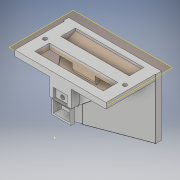
# Autodesk Inventor part: ventilador controladora
Saved by Autodesk Inventor 2019 (Build 230136000, 136)
## iProperties
Created: 2018-08-15
Part Number: ventilador controladora
Material: Genérico
Document SubType Name: Modeling
Designer: Albert Garangou Culebras
Density: 1 g/cm^3
Appearance: Valor por defecto
Author: Albert Garangou Culebras
Autodesk Inventor part; units mm, degrees
sketch "Boceto1" plane through (0, 0, 0) normal (0, 0, 1) x (1, 0, 0)
  line L0 (0, 0) -> (16, 0)
  line L1 (16, 0) -> (16, -12)
  line L2 (16, -12) -> (0, -12)
  line L3 (0, -12) -> (0, 0)
  line L4 (1, -1) -> (15, -1)
  line L5 (15, -1) -> (15, -11)
  line L6 (15, -11) -> (1, -11)
  line L7 (1, -11) -> (1, -1)
  dimension "d0" = 16
  dimension "d1" = 12
  constraints: 16 end point, 4 parallel, 2 horizontal, 2 perpendicular
  measures "d0" distance of L1.end L2.end
  measures "d1" distance of L0.end L1.end
ref_plane "Plano de trabajo3" through (0, 0, -40) normal (0, 0, -1) x (-1, 0, 0)
sketch "Boceto4" plane through (0, 0, -40) normal (0, 0, -1) x (-1, 0, 0)
  line L0 (0, -12) -> (0, 0) projected
  line L1 (0, -6) -> (-16, -6)
  line L2 (-8, -31) -> (-48, -31)
  line L3 (-8, -31) -> (32, -31)
  line L4 (32, -31) -> (32, 19)
  line L5 (32, 19) -> (-48, 19)
  line L6 (-48, 19) -> (-48, -31)
  dimension "d8" = 40
  dimension "d9" = 40
  dimension "d10" = 80
  constraints: 12 end point, 2 horizontal, 1 midpoint, 1 perpendicular, 1 vertical
  measures "d8" distance of L2.start L2.end
  measures "d9" distance of L2.start L3.end
  measures "d10" distance of L4.end L5.end
extrude "Extrusión2" add sketch "Boceto1" against normal blind 40
loft "Solevación1" add profiles "Boceto4" section 1 edges at (1, -6, 0) (8, -1, 0) (15, -6, 0) (8, -11, 0)
sketch "Boceto5" plane through (0, 0, -40) normal (0, 0, -1) x (-1, 0, 0)
  line L0 (30, -29) -> (-46, -29)
  line L1 (-46, -29) -> (-46, 17)
  line L2 (-46, 17) -> (30, 17)
  line L3 (30, 17) -> (30, -29)
  point P0 (0, 0)
  constraints: 8 end point, 2 parallel, 1 horizontal, 1 perpendicular
sketch "Boceto6" plane through (0, 0, 0) normal (0, 0, 1) x (1, 0, 0)
  line L0 (1, -11) -> (15, -11)
  line L1 (15, -11) -> (15, -1)
  line L2 (15, -1) -> (1, -1)
  line L3 (1, -1) -> (1, -11)
  point P0 (0, 0)
  constraints: 8 end point, 2 parallel, 1 horizontal, 1 perpendicular
loft "Solevación2" cut profiles "Boceto6", "Boceto5"
sketch "Boceto7" plane through (0, 0, 0) normal (0, 0, 1) x (1, 0, 0)
  line L0 (0, 0) -> (16, 0) projected
  line L1 (16, -12) -> (0, -12) projected
  line L2 (0, 0) -> (16, 0)
  line L3 (16, 0) -> (16, -12)
  line L4 (16, -12) -> (0, -12)
  line L5 (0, -12) -> (0, 0)
  line L6 (1, -11) -> (1, -1) projected
  line L7 (1, -1) -> (15, -1)
  line L8 (15, -1) -> (15, -11)
  line L9 (15, -11) -> (1, -11)
  line L10 (1, -11) -> (1, -1)
  constraints: 16 end point, 4 parallel, 2 horizontal, 2 perpendicular
extrude "Extrusión3" add sketch "Boceto7" against normal blind 5
sketch "Boceto8" plane through (0, 0, 0) normal (0, 0, 1) x (1, 0, 0)
  line L0 (0, 0) -> (16, 0)
  line L1 (16, 0) -> (16, -12)
  line L2 (16, -12) -> (0, -12)
  line L3 (0, -12) -> (0, 0)
  line L4 (15, -1) -> (15, -11) projected
  line L5 (1, -1) -> (15, -1)
  line L6 (15, -1) -> (15, -11)
  line L7 (15, -11) -> (1, -11)
  line L8 (1, -11) -> (1, -1)
  constraints: 16 end point, 4 parallel, 2 horizontal, 2 perpendicular
extrude "Extrusión4" add sketch "Boceto8" along normal blind 3
ref_plane "Plano de trabajo7" through (-19.527, -29, -48.1166) normal (0.7904151, 0, -0.6125717) x (-0.6125717, 0, -0.7904151)
sketch "Boceto17" plane through (-19.527, -29, -48.1166) normal (0.7904151, 0, -0.6125717) x (-0.6125717, 0, -0.7904151)
  line L0 (-46.5554, 46) -> (0, 46) projected
  line L1 (-10.2918, 46) -> (-10.2918, 0)
  line L2 (-10.2918, 0) -> (-38.5761, 10)
  line L3 (-38.5761, 10) -> (-38, 37)
  line L4 (-38, 37) -> (-10.2918, 46)
  point P0 (-49.9938, 29)
  dimension "d37" = 30
  constraints: 8 end point, 1 point on line, 1 vertical
  measures "d37" distance of L1.end L2.end
ref_plane "Plano de trabajo8" through (35.7246, -29, -47.9634) normal (-0.7904151, 0, -0.6125717) x (-0.6125717, 0, 0.7904151)
sketch "Boceto18" plane through (35.7246, -29, -47.9634) normal (-0.7904151, 0, -0.6125717) x (-0.6125717, 0, 0.7904151)
  line L0 (0, 46) -> (46.5554, 46) projected
  line L1 (10.0792, 46) -> (10.0792, 0)
  line L2 (46.5554, 0) -> (0, 0) projected
  line L3 (10.0792, 0) -> (38.3635, 10)
  line L4 (38.3635, 10) -> (38.3635, 36)
  line L5 (38.3635, 36) -> (10.0792, 46)
  point P0 (59.7949, 29)
  dimension "d39" = 30
  constraints: 8 end point, 2 point on line, 2 vertical
  measures "d39" distance of L1.end L3.end
extrude "Extrusión9" add sketch "Boceto18" along normal blind 0.8
extrude "Extrusión10" add sketch "Boceto17" along normal blind 0.8
ref_plane "Plano de trabajo9" through (0, 19, -2) normal (0, 1, 0) x (1, 0, 0)
sketch "Boceto22" plane through (0, 19, -2) normal (0, 1, 0) x (1, 0, 0)
  line L0 (-13.199, 38) -> (-30, 38) projected
  line L1 (-30, 38) -> (13, 38) construction
  line L2 (16, -0.7879) -> (48, 38) projected
  line L3 (48, 38) -> (48, -5)
  line L4 (48, 38) -> (91, 38) construction
  line L5 (48, -5) -> (-31.7513, -5)
  line L6 (48, 38) -> (-32, 38) projected
  line L7 (-31.7513, 38) -> (-31.7513, -5)
  line L8 (-31.7513, 38) -> (11.2487, 38) construction
  line L9 (-31.7513, -5) -> (-21.7513, -5)
  line L10 (-21.7513, -5) -> (-21.7513, 38)
  line L11 (-21.7513, 38) -> (-31.7513, 38)
  line L12 (48, -5) -> (38, -5)
  line L13 (38, -5) -> (38, 38)
  line L14 (48, 38) -> (38, 38)
  point P0 (0, -2)
  dimension "d46" = 90
  dimension "d47" = 43
  dimension "d49" = 90
  dimension "d50" = 10
  dimension "d51" = 43
  dimension "d52" = 90
  dimension "d53" = 10
  dimension "d54" = 43
  constraints: 24 end point, 4 perpendicular, 4 point on line, 3 horizontal, 1 collinear
  measures "d46" angle of L3 L4
  measures "d47" distance of L2.end L3.end
  measures "d49" angle of L7 L8
  measures "d50" distance of L5.end L9.end
  measures "d51" distance of L9.end L10.end
  measures "d52" angle of L10 L9
  measures "d53" distance of L3.end L12.end
  measures "d54" distance of L12.end L13.end
extrude "Extrusión11" add sketch "Boceto22" against normal blind 3 contours L10 L5 L7 L6 L0 | L6 L2 L13 | L3 L5 L13 L2
sketch "Boceto24" plane through (38, 19, -40) normal (-1, 0, 0) x (0, 0, 1)
  line L0 (0, 0) -> (43, 0) projected
  line L1 (35.5, -2) -> (35.5, 0)
  line L2 (35.5, 0) -> (43, 0)
  line L3 (43, 0) -> (43, -2)
  line L4 (35.5, -2) -> (35.5, -3)
  line L5 (43, -3) -> (6, -3) projected
  line L6 (43, -3) -> (35.5, -3)
  line L7 (43, -3) -> (43, -2)
  line L8 (43, 0) -> (43, -3) projected
  point P0 (40, -19)
  dimension "d57" = 7.5
  constraints: 12 end point, 2 collinear, 2 point on line, 1 parallel, 1 vertical
  measures "d57" distance of L1.end L2.end
extrude "Extrusión12" add sketch "Boceto24" along normal blind 60
sketch "Boceto25" plane through (-31.7513, 19, 3) normal (0, 0, 1) x (1, 0, 0)
  line L0 (79.7513, -3) -> (0, -3) projected
  line L1 (39.8756, -3) -> (49.3756, -3)
  line L2 (39.8756, -3) -> (30.3756, -3)
  line L3 (30.3756, -3) -> (30.3756, -19)
  line L4 (30.3756, -19) -> (49.3756, -19)
  line L5 (49.3756, -19) -> (49.3756, -3)
  point P0 (31.7513, -19)
  dimension "d60" = 9.5
  dimension "d61" = 9.5
  dimension "d63" = 16
  dimension "d64" = 19
  constraints: 10 end point, 2 perpendicular, 2 point on line, 1 midpoint
  measures "d60" distance of L1.start L1.end
  measures "d61" distance of L1.start L2.end
  measures "d63" distance of L2.end L3.end
  measures "d64" distance of L3.end L4.end
extrude "Extrusión13" add sketch "Boceto25" against normal blind 7.5
sketch "Boceto27" plane through (0, 0, -40) normal (0, 0, -1) x (-1, 0, 0)
  line L0 (31.7513, 19) -> (-48, 19) projected
  line L1 (31.7513, 19) -> (-48, 19)
  line L2 (-48, 19) -> (-48, -31)
  line L3 (-48, -31) -> (31.7513, -31)
  line L4 (31.7513, -31) -> (31.7513, 19)
  line L5 (30, 16) -> (30, -29) projected
  line L6 (-46, -29) -> (-46, 16) projected
  line L7 (30, 17) -> (-46, 17)
  line L8 (-46, 17) -> (-46, -29)
  line L9 (-46, -29) -> (30, -29)
  line L10 (30, -29) -> (30, 17)
  point P0 (0, 0)
  constraints: 16 end point, 4 parallel, 2 horizontal, 2 perpendicular
extrude "Extrusión15" add sketch "Boceto27" along normal blind 5
sketch "Boceto28" plane through (0, -12, -2) normal (0, -1, 0) x (1, 0, 0)
  line L0 (16, 1) -> (0, 1)
  line L1 (0, 1) -> (0, 5)
  line L2 (0, 5) -> (16, 5)
  line L3 (16, 5) -> (16, 1)
  point P0 (0, 2)
  constraints: 8 end point, 2 parallel, 1 horizontal, 1 perpendicular
extrude "Extrusión16" add sketch "Boceto28" against normal blind 12
sketch "Boceto30" plane through (0, 0, 3) normal (0, 0, 1) x (1, 0, 0)
  line L0 (15, -11) -> (1, -11)
  line L1 (1, -11) -> (1, -1)
  line L2 (1, -1) -> (15, -1)
  line L3 (15, -1) -> (15, -11)
  point P0 (0, 0)
  constraints: 8 end point, 2 parallel, 1 horizontal, 1 perpendicular
extrude "Extrusión17" cut sketch "Boceto30" against normal blind 7.75
sketch "Boceto31" plane through (-32, -31, -40) normal (-0.7713733, 0, 0.636383) x (0.636383, 0, 0.7713733)
  line L0 (50.2239, 30.5806) -> (50.2239, 19.4194) projected
  line L1 (50.2239, 30.5806) -> (50.2239, 19.4194)
  line L2 (50.2239, 19.4194) -> (36, 14)
  line L3 (36, 14) -> (36, 36.1153)
  line L4 (50.2842, 30.6061) -> (7.7783, 47) projected
  line L5 (50.2239, 30.5806) -> (36, 36.1153)
  point P0 (51.2192, 31)
  constraints: 8 end point, 1 collinear, 1 parallel, 1 point on line
extrude "Extrusión18" add sketch "Boceto31" against normal blind 1
sketch "Boceto32" plane through (16, -11.6061, -1.2121) normal (0.7713733, 0, 0.636383) x (0.636383, 0, -0.7713733)
  line L0 (0.0603, 11.1867) -> (0.7792, 11.6061) projected
  line L1 (0.0603, -0.0001) -> (0.0603, 11.1867)
  line L2 (0.0603, 11.1867) -> (9.1306, 14.7337)
  line L3 (0, 11.2121) -> (42.5059, 27.6061) projected
  line L4 (9.1306, -0.0002) -> (9.1306, 14.7337)
  line L5 (-0.6264, 30.6061) -> (-0.6264, -19.3939) projected
  line L6 (9.1306, -0.0002) -> (9.1306, -3.5355)
  line L7 (9.1306, -3.5355) -> (0.0603, -0.0003)
  line L8 (0.0603, 0.0254) -> (0.0603, 11.1867) projected
  line L9 (0.0603, -0.0003) -> (0.0603, 11.1867)
  point P0 (-11.1171, 11.6061)
  constraints: 12 end point, 2 vertical, 1 collinear, 1 parallel, 1 point on line
extrude "Extrusión19" add sketch "Boceto32" against normal blind 1 contours L2 L4 L6 L7 L1
sketch "Boceto33" plane through (0, -12, -2) normal (0, -0.8944272, 0.4472136) x (1, 0, 0)
  line L0 (0, -0.7008) -> (0, 4.6658) projected
  line L1 (0, 0.8542) -> (-9.5417, -11.818)
  line L2 (-8.3188, -11.8619) -> (-4.3774, -6.6273) projected
  line L3 (-9.5417, -11.818) -> (25.3705, -11.818)
  line L4 (11.5919, -17.558) -> (11.5919, -5.9304) projected
  line L5 (16, 0.8809) -> (19.6301, -4.0385) projected
  line L6 (25.3705, -11.818) -> (16, 0.8809)
  line L7 (16, 4.4721) -> (16, 0) projected
  line L8 (16, 0.8809) -> (16, 0)
  line L9 (16, 0) -> (0, 0)
  line L10 (0, 0) -> (0, 0.8542)
  line L11 (0, 4.4721) -> (0, 0) projected
  point P0 (0, 7.1554)
  point P1 (0, 0.0965)
  point P2 (0, 5.2759)
  constraints: 12 end point, 3 point on line, 2 collinear, 1 parallel, 1 perpendicular
extrude "Extrusión20" add sketch "Boceto33" against normal blind 1
sketch "Boceto34" plane through (0, 0, -2) normal (0, 0.8944272, 0.4472136) x (1, 0, 0)
  line L0 (30.35, 18.5661) -> (-13.525, 17.4481)
  line L1 (0, -0.8809) -> (-27.05, 35.7771) projected
  line L2 (-13.525, 17.4481) -> (0.825, -1.9989)
  line L3 (0.825, -1.9989) -> (0, -0.0364)
  line L4 (0, 0) -> (0, -0.8809) projected
  line L5 (0, 0) -> (16, 0)
  line L6 (16, 0) -> (0, 0) projected
  line L7 (16, -0.8809) -> (16, 0) projected
  line L8 (16, 0) -> (16, -0.8809)
  line L9 (16, -0.8809) -> (30.35, 18.5661)
  line L10 (16, -0.8809) -> (43.05, 35.7771) projected
  point P0 (0, -1.7889)
  point P1 (17.6244, 2.2361)
  point P2 (17.6244, 2.7951)
  constraints: 12 end point, 2 collinear, 1 midpoint, 2 other
extrude "Extrusión21" [suppressed]
sketch "Boceto35" plane through (16, -11.6061, -1.2121) normal (0.7713733, 0, 0.636383) x (0.636383, 0, -0.7713733)
  line L0 (0, 0) -> (16, -6.171)
  line L1 (9.1306, -3.5216) -> (50.2842, -19.3939) projected
  line L2 (16, -6.171) -> (16, 17.3831)
  line L3 (0, 11.2121) -> (42.5059, 27.6061) projected
  line L4 (0, 0) -> (0, 11.2121) projected
  line L5 (0, 11.2121) -> (16, 17.3831)
  line L6 (0, 11.2121) -> (0.6077, 11.6061) projected
  line L7 (0, 11.2121) -> (0, 0)
  line L8 (1.2121, 11.6061) -> (1.2121, 0.3323) projected
  point P0 (-11.1171, 11.6061)
  point P1 (1.2121, 10.8798)
  point P2 (1.2121, 0.3323)
  point P3 (0.303, 10.4264)
  point P4 (0.303, 0.7857)
  constraints: 8 end point, 2 point on line, 2 vertical, 1 other
extrude "Extrusión22" add sketch "Boceto35" against normal blind 1
sketch "Boceto37" plane through (0, 0, 3) normal (0, 0, 1) x (1, 0, 0)
  line L0 (0, -12) -> (16, -12) projected
  line L1 (0, -12) -> (16, -12)
  line L2 (16, -12) -> (16, 0)
  line L3 (16, 0) -> (0, 0)
  line L4 (0, 0) -> (0, -12)
  line L5 (1, -1) -> (15, -1) projected
  line L6 (15, -1) -> (1, -1)
  line L7 (1, -1) -> (1, -11)
  line L8 (1, -11) -> (15, -11)
  line L9 (15, -11) -> (15, -1)
  constraints: 16 end point, 4 parallel, 2 horizontal, 2 perpendicular
extrude "Extrusión23" cut sketch "Boceto37" against normal blind 1
sketch "Boceto38" plane through (-31.7513, 19, 3) normal (0, 0, 1) x (1, 0, 0)
  line L0 (30.3756, -17.75) -> (49.3756, -17.75) projected
  line L1 (30.3756, -19) -> (49.3756, -19) projected
  line L2 (39.8756, -19) -> (39.8756, -14)
  line L3 (39.8756, -14) -> (39.8756, -15)
  circle A0 centre (39.8756, -15) radius 1.75
  point P0 (31.7513, -19)
  dimension "d94" = 5
  dimension "d146" = 1
  dimension "d147" = 3.5
  constraints: 4 end point, 2 coincident, 1 centre point, 1 midpoint, 1 point on line
  measures "d94" distance of L2.start L2.end
  measures "d146" distance of L3.start L3.end
  measures "d147" diameter of A0
extrude "Extrusión24" cut sketch "Boceto38" against normal blind 7.75
sketch "Boceto39" plane through (-31.7513, 19, 3) normal (0, 0, 1) x (1, 0, 0)
  line L0 (34.4248, -19) -> (45.4248, -19)
  line L1 (45.4248, -9.5) -> (45.6748, -9.5)
  line L2 (45.6748, -9.5) -> (45.6748, -19)
  line L3 (16.8005, -9.5) -> (16.5505, -9.5)
  line L4 (45.6748, -19) -> (33.6748, -19)
  line L5 (45.4248, -9.5) -> (33.6748, -9.5)
  line L6 (33.6748, -19) -> (33.6748, -9.5)
  line L7 (30.3756, -17.75) -> (49.3756, -17.75) projected
  point P0 (30.3756, -3)
  point P1 (49.3756, -3)
  point P2 (16.5505, -19)
  dimension "d100" = 9.5
  dimension "d103" = 0.25
  dimension "d104" = 0.25
  dimension "d109" = 12
  constraints: 14 end point, 2 perpendicular, 1 horizontal
  measures "d100" distance of L0.end L1.start
  measures "d103" distance of L1.start L1.end
  measures "d104" distance of L3.start L3.end
  measures "d109" distance of L2.end L4.end
extrude "Extrusión25" cut sketch "Boceto39" against normal blind 2
sketch "Boceto40" plane through (0, 16, -2) normal (0, -1, 0) x (1, 0, 0)
  line L0 (-31.7513, -38) -> (-31.7513, 5) projected
  line L1 (-31.7513, 5) -> (-31.7513, -38)
  line L2 (-31.7513, -16.5) -> (-22, -16.5)
  circle A0 centre (-26.8756, -16.5) radius 1.65
  circle A1 centre (43, -16.5) radius 1.65
  point P0 (0, 2)
  dimension "d105" = 3.3
  dimension "d106" = 3.3
  constraints: 4 end point, 2 centre point, 2 midpoint, 1 collinear, 1 horizontal
  measures "d105" diameter of A0
  measures "d106" diameter of A1
extrude "Extrusión26" cut sketch "Boceto40" against normal blind 38.5
sketch "Boceto41" plane through (0, 16, -2) normal (0, -1, 0) x (1, 0, 0)
  line L0 (38, -35.7778) -> (38, -38) projected
  line L1 (38, -35.7778) -> (38, -38)
  line L2 (38, -38) -> (46, -38) projected
  line L3 (38, -38) -> (46, -38)
  line L4 (46, -38) -> (44.2885, -35.7778)
  line L5 (44.2885, -35.7778) -> (38, -35.7778)
  line L6 (-21.7513, -2.5) -> (-21.7513, -38) projected
  line L7 (-21.7513, -35.7778) -> (-21.7513, -38)
  line L8 (-30, -38) -> (-21.7513, -38) projected
  line L9 (-21.7513, -38) -> (-30, -38)
  line L10 (-30, -38) -> (-28.2778, -35.7778) projected
  line L11 (-30, -38) -> (-28.2778, -35.7778)
  line L12 (-28.2778, -35.7778) -> (-21.7513, -35.7778) projected
  line L13 (-28.2778, -35.7778) -> (-21.7513, -35.7778)
  point P0 (0, 2)
  constraints: 16 end point, 4 collinear, 2 parallel, 1 perpendicular, 1 point on line
extrude "Extrusión27" cut sketch "Boceto41" against normal blind 1
sketch "Boceto42" plane through (38, 16, -37.7778) normal (1, 0, 0) x (0, 0, -1)
  line L0 (2.2222, 1) -> (0, 1) projected
  line L1 (0, 0) -> (0, 1) projected
  line L2 (2.2222, 1) -> (0, 0)
  line L3 (0, 0) -> (0, 1)
  line L4 (0, 1) -> (2.2222, 1)
  point P0 (-37.7778, -16)
  constraints: 6 end point, 1 collinear, 1 perpendicular
sketch "Boceto43" plane through (-21.7513, 16, -37.7778) normal (-1, 0, 0) x (0, 0, 1)
  line L0 (0, 0) -> (-2.2222, 1) projected
  line L1 (-2.2222, 1) -> (0, 0)
  line L2 (0, 0) -> (0, 1) projected
  line L3 (0, 0) -> (0, 1)
  line L4 (0, 1) -> (-2.2222, 1)
  point P0 (37.7778, -16)
  constraints: 6 end point, 2 collinear, 1 perpendicular
extrude "Extrusión29" add sketch "Boceto43" along normal blind 8.75
extrude "Extrusión30" add sketch "Boceto42" along normal blind 8.25
sketch "Boceto44" plane through (0, 0, 3) normal (0, 0, 1) x (1, 0, 0)
  line L0 (13.9235, 0) -> (17.6244, 0) projected
  line L1 (17.6244, 0) -> (17.6244, 1)
  line L2 (17.6244, 1.25) -> (17.6244, 0.5905) projected
  line L3 (17.6244, 1.025) -> (-1.3756, 1.025) projected
  line L4 (17.6244, 1) -> (-1.3756, 1.025)
  line L5 (-1.3756, 1.025) -> (-1.377, 0.025)
  line L6 (-1.377, 0.025) -> (17.6244, 0)
  point P0 (0, 0)
  dimension "d118" = 1
  constraints: 8 end point, 2 perpendicular, 1 point on line
  measures "d118" distance of L0.end L1.end
extrude "Extrusión31" cut sketch "Boceto44" against normal blind 7.25 contours L6 L5 L4 L1
sketch "Boceto45" plane through (-0.65, 0, -2) normal (0, -1, 0) x (1, 0, 0)
  line L0 (-0.7256, 5) -> (2.5735, 5) projected
  line L1 (2.5735, 5) -> (-0.7256, 5)
  line L2 (-0.7256, 5) -> (-0.7256, -0.8796) projected
  line L3 (-0.7256, 5) -> (-0.7256, -0.8796)
  line L4 (0.65, 0) -> (0.65, 0.7879) projected
  line L5 (-0.7256, -0.8796) -> (0.65, 0)
  line L6 (0.65, 0) -> (0.65, 4)
  line L7 (0.65, 4) -> (2.5735, 4)
  line L8 (2.5735, 4) -> (2.5735, 5) projected
  line L9 (2.5735, 4) -> (2.5735, 5)
  line L10 (14.5735, 5) -> (18.2744, 5) projected
  line L11 (14.5735, 5) -> (18.2744, 5) projected
  line L12 (18.2744, 5) -> (14.5735, 5)
  line L13 (2.5735, 4) -> (14.5735, 4) projected
  line L14 (14.5735, 5) -> (14.5735, 4)
  line L15 (14.5735, 4) -> (16.65, 4)
  line L16 (16.65, 0.7879) -> (16.65, 0) projected
  line L17 (16.65, 4) -> (16.65, 0.7879)
  line L18 (18.2744, -1.181) -> (17.3, 0) projected
  line L19 (16.65, 0.7879) -> (18.2744, -1.181)
  line L20 (18.2744, 5) -> (18.2744, -1.181) projected
  line L21 (18.2744, -1.181) -> (18.2744, 5)
  line L22 (18.2744, 5) -> (14.5735, 5)
  point P0 (0.65, 2)
  constraints: 26 end point, 7 perpendicular, 3 collinear, 1 horizontal, 1 parallel
extrude "Extrusión32" cut sketch "Boceto45" against normal blind 0.5
sketch "Boceto46" plane through (-21.7513, 19, -4.5) normal (1, 0, 0) x (0, 0, -1)
  line L0 (35.5, 0) -> (29.5, -3) projected
  line L1 (0, 0) -> (35.5, 0) projected
  line L2 (35.5, 0) -> (0, 0)
  line L3 (17.75, 0) -> (22.75, 0)
  line L4 (22.75, 0) -> (12.75, 0)
  line L5 (22.75, 0) -> (22.75, -3)
  line L6 (-7.5, -3) -> (35.1985, -3) projected
  line L7 (22.75, -3) -> (12.75, -3)
  line L8 (15.65, -3) -> (12.35, -3) projected
  line L9 (29.5, -3) -> (0, -3) projected
  line L10 (12.75, -3) -> (12.75, 0)
  point P0 (-4.5, -19)
  dimension "d123" = 5
  dimension "d124" = 10
  constraints: 12 end point, 4 point on line, 1 collinear, 1 midpoint, 1 perpendicular, 1 vertical
  measures "d123" distance of L3.start L3.end
  measures "d124" distance of L3.end L4.end
extrude "Extrusión33" add sketch "Boceto46" along normal blind 61.5 contours L5 L6 L10 L1
sketch "Boceto47" plane through (0, 16, -2) normal (0, -1, 0) x (1, 0, 0)
  line L0 (38, -15.25) -> (38, -2.5) projected
  line L1 (-21.7513, -15.25) -> (38, -15.25) projected
  line L2 (38, -15.25) -> (-21.7513, -15.25)
  line L3 (-21.7513, -32) -> (-21.7513, -25.25) projected
  line L4 (-21.7513, -15.25) -> (-21.7513, -25.25)
  line L5 (-21.7513, -25.25) -> (38, -25.25) projected
  line L6 (-21.7513, -25.25) -> (38, -25.25)
  line L7 (38, -25.25) -> (38, -15.25)
  line L8 (-21.7513, -15.25) -> (-21.7513, -2.5) projected
  line L9 (-21.7513, -15.25) -> (-21.7513, -25.25)
  line L10 (8.1244, -15.25) -> (-1.8756, -15.25)
  line L11 (-1.8756, -15.25) -> (18.1244, -15.25)
  line L12 (18.1244, -15.25) -> (18.1244, -25.25)
  line L13 (-1.8756, -15.25) -> (-1.8756, -25.25)
  line L14 (18.1244, -25.25) -> (-1.8756, -25.25)
  point P0 (0, 2)
  dimension "d127" = 10
  dimension "d128" = 20
  constraints: 20 end point, 5 perpendicular, 4 point on line, 3 collinear, 1 midpoint
  measures "d127" distance of L10.start L10.end
  measures "d128" distance of L10.end L11.end
extrude "Extrusión34" add sketch "Boceto47" along normal blind 4.5 contours L1 L12 L5 L13
sketch "Boceto48" plane through (-21.7513, 19, -40) normal (0, 0.8944272, 0.4472136) x (1, 0, 0)
  line L0 (19.8756, -23.7023) -> (19.8756, -16.7705) projected
  line L1 (19.8756, -23.7023) -> (39.8756, -23.7023)
  line L2 (39.8756, -23.7023) -> (39.8756, -14.7023)
  line L3 (39.8756, -14.7023) -> (19.8756, -14.7023)
  line L4 (19.8756, -16.7705) -> (19.8756, -14.2549) projected
  line L5 (39.8756, -14.7023) -> (19.8756, -14.7023)
  point P0 (21.7513, -44.2741)
  dimension "d131" = 9
  constraints: 8 end point, 2 perpendicular, 1 collinear, 1 horizontal, 1 point on line
  measures "d131" distance of L1.end L2.end
extrude "Extrusión35" add sketch "Boceto48" along normal blind 7.25
sketch "Boceto49" plane through (0, 16, -2) normal (0, -1, 0) x (1, 0, 0)
  line L0 (-21.7513, -15.25) -> (-21.7513, -2.5) projected
  line L1 (-21.7513, -15.25) -> (-21.7513, -2.5)
  line L2 (38, -2.5) -> (17.6244, -2.5) projected
  line L3 (-21.7513, -2.5) -> (38, -2.5)
  line L4 (38, -2.5) -> (38, -15.25) projected
  line L5 (38, -2.5) -> (38, -15.25)
  line L6 (-21.7513, -15.25) -> (-1.8756, -15.25) projected
  line L7 (38, -15.25) -> (-21.7513, -15.25)
  point P0 (0, 2)
  constraints: 8 end point, 2 collinear, 1 perpendicular
extrude "Extrusión36" cut sketch "Boceto49" along normal blind 5.25
sketch "Boceto50" plane through (0, 19, -2) normal (0, 1, 0) x (1, 0, 0)
  line L0 (48, -5) -> (48, 43) projected
  line L1 (-31.7513, 43) -> (48, 43) projected
  line L2 (48, -5) -> (-31.7513, -5)
  line L3 (-31.7513, -5) -> (-31.7513, 43)
  line L4 (-31.7513, 43) -> (48, 43)
  line L5 (48, 43) -> (48, -5)
  line L6 (38, 2.5) -> (38, 15.25) projected
  line L7 (-21.7513, 15.25) -> (-21.7513, 2.5) projected
  line L8 (38, 2.5) -> (-21.7513, 2.5)
  line L9 (-21.7513, 2.5) -> (-21.7513, 15.25)
  line L10 (-21.7513, 15.25) -> (38, 15.25)
  line L11 (38, 15.25) -> (38, 2.5)
  line L12 (18.1244, 25.25) -> (38, 25.25) projected
  line L13 (-21.7513, 25.25) -> (-21.7513, 38) projected
  line L14 (38, 25.25) -> (-21.7513, 25.25)
  line L15 (-21.7513, 25.25) -> (-21.7513, 38)
  line L16 (-21.7513, 38) -> (38, 38)
  line L17 (38, 38) -> (38, 25.25)
  circle A0 centre (43, 16.5) radius 1.65 projected
  circle A1 centre (43, 16.5) radius 1.65
  circle A2 centre (-26.8756, 16.5) radius 1.65 projected
  circle A3 centre (-26.8756, 16.5) radius 1.65
  point P0 (0, -2)
  constraints: 24 end point, 6 parallel, 3 horizontal, 3 perpendicular, 2 centre point, 2 coincident
extrude "Extrusión37" add sketch "Boceto50" along normal blind 2
sketch "Boceto51" plane through (0, 0, 2) normal (0, 0, 1) x (1, 0, 0)
  line L0 (15, -0.4884) -> (0, -0.4884)
  line L1 (0, -0.4884) -> (0, 0.4536)
  line L2 (0, -12) -> (0, 0.0232) projected
  line L3 (0, 0.4536) -> (16.2563, 0.4536)
  line L4 (16.2563, 0.4536) -> (16.2563, -0.4884)
  line L5 (16.2563, -0.4884) -> (15, -0.4884)
  point P0 (0, 0)
  point P1 (0, -0.4194)
  point P2 (16, 0)
  point P3 (16, -0.3939)
  constraints: 10 end point, 2 collinear, 2 perpendicular, 1 horizontal, 1 point on line
extrude "Extrusión38" cut sketch "Boceto51" against normal blind 4.75
sketch "Boceto52" plane through (16, -12, 2) normal (1, 0, 0) x (0, 0, -1)
  line L0 (0, 0) -> (0, 11.5116) projected
  line L1 (0, 0) -> (0, 11.5116)
  line L2 (3.2121, 11.5116) -> (0, 11.5116) projected
  line L3 (0, 11.5116) -> (3.2121, 11.5116)
  line L4 (3.2121, 11.5116) -> (3.2121, 0)
  line L5 (3.2121, 11.5116) -> (3.2121, 0.3939) projected
  line L6 (0, 0) -> (4, 0) projected
  line L7 (3.2121, 0) -> (0, 0)
  point P0 (2, 12)
  constraints: 8 end point, 3 collinear, 1 vertical
extrude "Extrusión39" add sketch "Boceto52" along normal blind 0.3
sketch "Boceto53" plane through (0, -12, -2) normal (-1, 0, 0) x (0, 0, 1)
  line L0 (4, 11.5116) -> (0.7879, 11.5116) projected
  line L1 (4, 11.5116) -> (0.7879, 11.5116)
  line L2 (0.7879, 11.5116) -> (0.7879, 0)
  line L3 (4, 0) -> (0, 0) projected
  line L4 (0.7879, 0) -> (4, 0)
  line L5 (4, 0) -> (4, 11.5116)
  point P0 (2, 12)
  constraints: 8 end point, 2 collinear, 2 perpendicular
extrude "Extrusión40" add sketch "Boceto53" along normal blind 0.3
sketch "Boceto54" plane through (0, -12, -2) normal (0, -1, 0) x (1, 0, 0)
  line L0 (16, 0.7879) -> (16.3, 0.7879) projected
  line L1 (16.3, 4) -> (16.3, 0.7879) projected
  line L2 (16.3, 0.7879) -> (16.3, 4)
  line L3 (16.3, 4) -> (-0.3, 4) projected
  line L4 (16.3, 4) -> (-0.3, 4)
  line L5 (-0.3, 0.7879) -> (-0.3, 4) projected
  line L6 (-0.3, 4) -> (-0.3, 0.7879)
  line L7 (-0.3, 0.7879) -> (16.3, 0.7879)
  point P0 (0, 2)
  constraints: 8 end point, 2 collinear, 2 perpendicular
extrude "Extrusión41" add sketch "Boceto54" along normal blind 0.75
sketch "Boceto55" plane through (48, -31, -40) normal (0.7713733, 0, 0.636383) x (0.636383, 0, -0.7713733)
  line L0 (0, 0) -> (0, 47) projected
  line L1 (0, 47) -> (0, 0)
  line L2 (-49.6764, 19) -> (-50.2842, 19.3939) projected
  line L3 (0, 0) -> (-50.2842, 19.3939)
  line L4 (-47.7317, 31.5905) -> (-7.7783, 47) projected
  line L5 (-50.2842, 30.5116) -> (-7.7783, 47)
  line L6 (-7.7783, 47) -> (0, 47)
  line L7 (-1.2728, 48) -> (2.5841, 48) projected
  line L8 (-50.2842, 19.3939) -> (-44.58, 17.1939) projected
  line L9 (-50.2842, 19.3939) -> (-45.6191, 17.5947)
  line L10 (-45.6191, 17.5947) -> (-45.0873, 17.3896)
  line L11 (-45.0873, 17.3896) -> (-45.0873, 32.5275)
  point P0 (-61.4013, 31)
  point P1 (-45.6191, 32.3212)
  dimension "d159" = 5
  dimension "d160" = 0.57
  constraints: 14 end point, 4 point on line, 1 collinear, 1 parallel, 1 vertical
  measures "d159" distance of L2.end L9.end
  measures "d160" distance of L9.end L10.end
extrude "Extrusión42" add sketch "Boceto55" along normal blind 0.4
sketch "Boceto56" plane through (-32, -31, -40) normal (-0.7713733, 0, 0.636383) x (0.636383, 0, 0.7713733)
  line L0 (50.2842, 19.3939) -> (49.6764, 19) projected
  line L1 (50.0933, 30.5116) -> (8.0419, 47)
  line L2 (7.7783, 47) -> (0.3908, 47) projected
  line L3 (8.0419, 47) -> (0.3908, 47)
  line L4 (0.3908, 47) -> (0.3908, 50)
  line L5 (0.3908, 49.8493) -> (0, 50) projected
  line L6 (0.3908, 50) -> (0, 50)
  line L7 (35.5595, 13.7148) -> (0, 0) projected
  line L8 (0, 50) -> (0, 0)
  line L9 (0, 0) -> (50.2842, 19.3939)
  line L10 (59.4432, 30.5116) -> (49.0979, 30.5116) projected
  line L11 (50.0933, 30.5116) -> (45.4383, 32.3368)
  line L12 (45.4383, 17.525) -> (45.2015, 17.4448)
  line L13 (48.7399, 18.7983) -> (35.4506, 13.7148) projected
  line L14 (45.2015, 17.4448) -> (44.968, 17.3555)
  line L15 (44.968, 17.3555) -> (45.1081, 17.4091)
  line L16 (45.1081, 17.4091) -> (45.1081, 32.4663)
  point P0 (51.2192, 31)
  point P1 (45.2015, 32.4297)
  dimension "d155" = 5
  dimension "d156" = 0.25
  dimension "d157" = 0.25
  dimension "d158" = 0.15
  constraints: 22 end point, 10 point on line, 3 perpendicular, 1 collinear, 1 vertical
  measures "d155" distance of L11.start L11.end
  measures "d156" distance of L12.start L12.end
  measures "d157" distance of L12.end L14.end
  measures "d158" distance of L14.end L15.end
extrude "Extrusión43" add sketch "Boceto56" along normal blind 0.4 contours L16 L13 L12 L9 L7 L8 L5 L4 L2 L3 L1
sketch "Boceto57" plane through (0, -12, -2) normal (0, -0.8944272, 0.4472136) x (1, 0, 0)
  line L0 (-31.7513, -42.4853) -> (48, -42.4853) projected
  line L1 (-31.7513, -42.4853) -> (-31.7513, -46.9574) projected
  line L2 (48, -42.4853) -> (-31.7513, -42.4853)
  line L3 (-31.7513, -42.4853) -> (-32, -42.4853)
  line L4 (-32, -42.4853) -> (-32.3085, -42.2576) projected
  line L5 (-32, -42.4853) -> (-1.3879, -1)
  line L6 (-3.0838, -3.2983) -> (-32, -42.4853) projected
  line L7 (-0.34, 0.4201) -> (-3.3088, -3.6031)
  line L8 (-3.3088, -3.6031) -> (19.3088, -3.6031)
  line L9 (19.3072, -3.601) -> (19.6301, -4.0385) projected
  line L10 (48, -42.4853) -> (48, -21.4663) projected
  line L11 (19.3088, -3.6031) -> (48, -42.4853)
  point P0 (0, 7.1554)
  point P1 (0, 0.8809)
  point P2 (16, 0.8809)
  point P3 (18.9688, -3.1424)
  dimension "d152" = 5
  constraints: 12 end point, 4 point on line, 2 horizontal, 1 perpendicular
  measures "d152" distance of L7.start L7.end
extrude "Extrusión44" add sketch "Boceto57" along normal blind 0.4
sketch "Boceto58" plane through (0, 0, -40) normal (0, 0, -1) x (-1, 0, 0)
  line L0 (32.3085, 19) -> (32.3085, -31) projected
  line L1 (31.7513, 19) -> (31.7513, -31) projected
  line L2 (32.3085, -31) -> (31.7513, -31)
  line L3 (31.7513, -31) -> (31.7513, 19)
  line L4 (31.7513, 19) -> (32.3085, 19)
  line L5 (32.3085, 19) -> (32.3085, -31)
  point P0 (0, 0)
  constraints: 8 end point, 2 parallel, 1 horizontal, 1 perpendicular
extrude "Extrusión45" add sketch "Boceto58" along normal blind 5
sketch "Boceto59" plane through (48, -31.3578, -39.8211) normal (0, -0.4472136, -0.8944272) x (-1, 0, 0)
  line L0 (0, 0) -> (28.6912, 0) projected
  line L1 (80.3085, 0.4) -> (80, 0.4) projected
  line L2 (0, 0) -> (80, 0)
  line L3 (80, 0) -> (80, 0.4)
  line L4 (80, 0.4) -> (0, 0.4)
  line L5 (0, 0.4) -> (0, 0)
  point P0 (48, 10.2387)
  constraints: 8 end point, 2 parallel, 1 horizontal, 1 perpendicular
sketch "Boceto60" plane through (48, -31, -45) normal (1, 0, 0) x (0, 0, -1)
  line L0 (-5, 2) -> (-5, 47) projected
  line L1 (-5, 0) -> (0, 0) projected
  line L2 (-5, 47) -> (0, 47)
  line L3 (0, 47) -> (0, 0)
  line L4 (0, 0) -> (-5, 0)
  line L5 (-5, 0) -> (-5, 47)
  point P0 (-45, 31)
  constraints: 8 end point, 2 parallel, 1 horizontal, 1 perpendicular
extrude "Extrusión46" add sketch "Boceto60" along normal blind 0.4
sketch "Boceto61" plane through (-32.3085, -31, -45) normal (0, -1, 0) x (1, 0, 0)
  point P0 (32.3085, 45)
sketch "Boceto62" plane through (-32.3085, -31, -39.7454) normal (0.2290022, -0.9330103, 0.2775784) x (0.7713733, 0, -0.636383)
  line L0 (0.2862, 48.3219) -> (0.2862, 0) projected
  line L1 (0.2862, 48.3219) -> (0, 48)
  line L2 (0, 53.7693) -> (0, 24.4161) projected
  line L3 (0, 17.9925) -> (0, 0) projected
  line L4 (0, 48) -> (0, 0)
  line L5 (0, 0) -> (0.2862, 0)
  line L6 (0.4, 0) -> (0, 0) projected
  line L7 (0.2862, 0) -> (61.996, 47.5001) projected
  line L8 (0.2862, 48.3219) -> (0.2862, 0)
  line L9 (0.2862, 0) -> (0, 0)
  point P0 (-0.3714, 58.9434)
  constraints: 10 end point, 2 point on line, 2 vertical, 1 perpendicular
extrude "Extrusión47" add sketch "Boceto62" along normal blind 0.38
sketch "Boceto63" plane through (-32.3085, -31, -45) normal (0, -1, 0) x (1, 0, 0)
  line L0 (0, 5) -> (0, 0) projected
  line L1 (80.7085, 5) -> (80.7085, 0) projected
  line L2 (0, 0) -> (80.7085, 0)
  line L3 (80.7085, 0) -> (80.7085, 5)
  line L4 (80.7085, 5) -> (0, 5)
  line L5 (0, 5) -> (0, 0)
  point P0 (32.3085, 45)
  constraints: 8 end point, 2 parallel, 1 horizontal, 1 perpendicular
extrude "Extrusión48" add sketch "Boceto63" along normal blind 0.5
sketch "Boceto64" plane through (-32.3085, 19, -45) normal (-1, 0, 0) x (0, 0, 1)
  line L0 (0, 0) -> (0, -50.5) projected
  line L1 (5, -50.5) -> (0, -50.5) projected
  line L2 (0, 0) -> (5, 0)
  line L3 (5, 0) -> (5, -50.5)
  line L4 (5, -50.5) -> (0, -50.5)
  line L5 (0, -50.5) -> (0, 0)
  point P0 (45, -19)
  constraints: 8 end point, 2 parallel, 1 horizontal, 1 perpendicular
extrude "Extrusión49" add sketch "Boceto64" along normal blind 0.3
sketch "Boceto65" plane through (-32, 19, -40) normal (0, 1, 0) x (1, 0, 0)
  line L0 (-0.6085, 0) -> (-0.6085, 5) projected
  line L1 (0.2487, 5) -> (0.2487, 0) projected
  line L2 (-0.6085, 5) -> (0.2487, 5)
  line L3 (0.2487, 5) -> (0.2487, 0)
  line L4 (0.2487, 0) -> (-0.6085, 0)
  line L5 (-0.6085, 0) -> (-0.6085, 5)
  line L6 (80, 0) -> (80, 5) projected
  line L7 (80.4, 5) -> (80.4, 0) projected
  line L8 (80, 5) -> (80.4, 5)
  line L9 (80.4, 5) -> (80.4, 0)
  line L10 (80.4, 0) -> (80, 0)
  line L11 (80, 0) -> (80, 5)
  point P0 (32, -40)
  constraints: 16 end point, 4 parallel, 2 horizontal, 2 perpendicular
extrude "Extrusión50" add sketch "Boceto65" along normal blind 2
sketch "Boceto66" plane through (48, 16, -40) normal (0, 1, 0) x (1, 0, 0)
  line L0 (0, 0) -> (0.4, 0) projected
  line L1 (0, 5) -> (0.4, 5)
  line L2 (0.4, 5) -> (0.4, 0)
  line L3 (0.4, 0) -> (0, 0)
  line L4 (0, 0) -> (0, 5)
  point P0 (-48, -40)
  constraints: 8 end point, 2 parallel, 1 horizontal, 1 perpendicular
extrude "Extrusión51" add sketch "Boceto66" along normal blind 3.25
